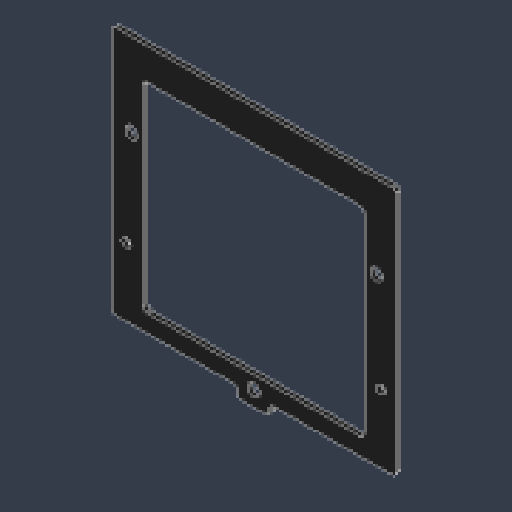
# Autodesk Inventor part: PlacementTest
Saved by Autodesk Inventor 2023.4 (Build 274418000, 418)
## iProperties
Created: 2024-02-22
Part Number: PlacementTest
Material: Generic
Document SubType Name: Modeling
Designer: JoaoSilva
Density: 1 g/cm^3
Appearance: Smooth - Black
Author: JoaoSilva
Autodesk Inventor part; units mm, degrees
ref_plane "YZ Plane" through (0, 0, 0) normal (1, 0, 0) x (0, 1, 0)
ref_plane "XZ Plane" through (0, 0, 0) normal (0, 1, 0) x (-1, 0, 0)
ref_plane "XY Plane" through (0, 0, 0) normal (0, 0, 1) x (1, 0, 0)
sketch "Sketch1" plane through (0, 0, 0) normal (0, 0, 1) x (1, 0, 0)
  line L0 (-40, 32.5) -> (40, 32.5)
  line L1 (40, 32.5) -> (40, -32.5)
  line L2 (40, -32.5) -> (-40, -32.5)
  line L3 (-40, -32.5) -> (-40, 32.5)
  line L4 (-40, 32.5) -> (40, -32.5) construction
  line L5 (40, 32.5) -> (-40, -32.5) construction
  line L6 (-8, 32.5) -> (-8, 24.5)
  line L7 (-8, 24.5) -> (-20, 24.5)
  line L8 (-20, 24.5) -> (-20, 28.5)
  line L9 (-20, 28.5) -> (-40, 28.5)
  line L10 (-40, -27) -> (-19, -27)
  line L11 (-19, -27) -> (-15.5, -23.5)
  line L12 (-15.5, -23.5) -> (-9.5, -23.5)
  line L13 (-9.5, -23.5) -> (-9.5, -32.5)
  line L14 (9.5, -32.5) -> (9.5, -23.5)
  line L15 (9.5, -23.5) -> (15.5, -23.5)
  line L16 (15.5, -23.5) -> (19, -27)
  line L17 (19, -27) -> (40, -27)
  point P0 (0, 0)
  dimension "d0" = 80
  dimension "d1" = 65
  dimension "d2" = 19
  dimension "d3" = 45
  dimension "d4" = 9
  dimension "d5" = 3.5
  dimension "d6" = 6
  dimension "d7" = 45
  dimension "d8" = 8
  dimension "d9" = 8
  dimension "d10" = 12
  dimension "d11" = 4
  constraints: 36 end point, 9 perpendicular, 6 point on line, 4 equal length, 3 parallel, 2 midpoint, 1 horizontal, 1 vertical
  measures "d0" distance of L1.end L2.end
  measures "d1" distance of L0.end L1.end
  measures "d2" distance between parallel lines of L14 L13
  measures "d3" angle of L10 L11
  measures "d4" distance of L12.end L13.end
  measures "d5" distance between parallel lines of L12 L10
  measures "d6" distance of L11.end L12.end
  measures "d7" angle of L17 L16
  measures "d8" distance from line of point (0, 0) L6
  measures "d9" distance of L6.start L6.end
  measures "d10" distance of L6.end L7.end
  measures "d11" distance between parallel lines of L7 L9
extrude "Extrusion1" add sketch "Sketch1" along normal blind 1.3 contours L0 L1 L17 L16 L15 L14 L2 L13 L12 L11 L10 L3 L9 L8 L7 L6
sketch "Sketch2" plane through (0, 0, 1.3) normal (0, 0, 1) x (1, 0, 0)
  line L0 (-35.7, -4.3) -> (35.7, -4.3) construction
  line L1 (-40, -27) -> (-19, -27) projected
  point P0 (0, 0)
  point P1 (0, -4.3)
  dimension "d14" = 71.4
  dimension "d15" = 22.7
  constraints: 2 end point, 1 horizontal, 1 midpoint, 1 vertical alignment
  measures "d14" distance of L0.start L0.end
  measures "d15" distance between parallel lines of L1 L0
hole "Hole1" at (-35.7, -4.3, 1.3) at (35.7, -4.3, 1.3) direction (0, 0, -1) diameter 2.5 end through all
sketch "Sketch4" plane through (-8, 32.5, 0) normal (0, 1, 0) x (1, 0, 0)
  line L0 (10.9, -2.9) -> (5.1, -2.9) construction
  line L1 (10.9, -1.3) -> (5.1, -1.3)
  line L2 (5.1, -4.5) -> (10.9, -4.5)
  arc A0 (10.9, -4.5) -> (10.9, -1.3) centre (10.9, -2.9) ccw
  arc A1 (5.1, -1.3) -> (5.1, -4.5) centre (5.1, -2.9) ccw
  line L3 (48, -1.3) -> (0, -1.3) projected
  line L4 (10.9, -2.9) -> (5.1, -2.9) construction
  line L5 (10.9, -1.7) -> (5.1, -1.7)
  line L6 (5.1, -4.1) -> (10.9, -4.1)
  arc A2 (10.9, -4.1) -> (10.9, -1.7) centre (10.9, -2.9) ccw
  arc A3 (5.1, -1.7) -> (5.1, -4.1) centre (5.1, -2.9) ccw
  point P0 (8, 0)
  point P1 (8, -2.9)
  point P2 (3.5, -2.9)
  point P3 (12.5, -2.9)
  point P4 (8, -2.9)
  dimension "d23" = 3.2
  dimension "d24" = 9
  dimension "d25" = 0.4
  constraints: 16 end point, 10 point on circle, 8 tangent, 4 centre point, 3 equal length, 2 midpoint, 1 collinear, 1 horizontal, 1 vertical alignment
  measures "d23" distance between parallel lines of L2 L1
  measures "d24" distance of point (3.5, -2.9) point (12.5, -2.9)
  measures "d25" distance between parallel lines of L2 L6
extrude "Extrusion2" add sketch "Sketch4" against normal blind 6.8
sketch "Sketch5" plane through (0, 0, 1.3) normal (0, 0, 1) x (1, 0, 0)
  circle A0 centre (-34.4, 23.1) radius 1.7
  circle A1 centre (34.4, 23.1) radius 1.7
  circle A2 centre (0, -22.3) radius 1.7
  line L0 (-34.4, 23.1) -> (34.4, 23.1) construction
  circle A3 centre (35.7, -4.3) radius 1.25 projected
  point P0 (0, 0)
  point P1 (0, 23.1)
  dimension "d28" = 3.4
  dimension "d29" = 68.8
  dimension "d30" = 27.4
  dimension "d31" = 18
  constraints: 3 centre point, 2 end point, 2 equal radius, 2 vertical alignment, 1 horizontal, 1 horizontal alignment, 1 midpoint
  measures "d28" diameter of A2
  measures "d29" distance of L0.start L0.end
  measures "d30" distance from line of A3.centre L0
  measures "d31" vertical distance of A3.centre A2.centre
extrude "Extrusion3" add sketch "Sketch5" along normal blind 0.4 contours A0 | A1 | A2
sketch "Sketch6" plane through (0, -22.3, 1.7) normal (0, 0, 1) x (1, 0, 0)
  circle A0 centre (0, 0) radius 1.7 projected
  circle A1 centre (-34.4, 45.4) radius 1.7 projected
  circle A2 centre (34.4, 45.4) radius 1.7 projected
  point P0 (0, 22.3)
extrude "Extrusion4" cut sketch "Sketch6" against normal through all
sketch "Sketch7" plane through (0, 0, 1.3) normal (0, 0, 1) x (1, 0, 0)
  line L0 (40, 32.5) -> (-8, 32.5) projected
  line L1 (40, 32.5) -> (40, 46.5)
  line L2 (40, 46.5) -> (-40, 46.5)
  line L3 (-40, 28.5) -> (-40, -27) projected
  line L4 (-40, 46.5) -> (-40, 28.5)
  line L5 (-40, 28.5) -> (-31, 28.5)
  line L6 (-20, 28.5) -> (-40, 28.5) projected
  line L7 (-31, 28.5) -> (-31, 37.5)
  line L8 (-31, 37.5) -> (31, 37.5)
  line L9 (31, 37.5) -> (31, 32.5)
  point P0 (0, 0)
  dimension "d36" = 9
  dimension "d37" = 9
  dimension "d38" = 9
  dimension "d39" = 5
  constraints: 14 end point, 4 perpendicular, 2 point on line, 2 vertical
  measures "d36" distance between parallel lines of L7 L4
  measures "d37" distance between parallel lines of L2 L8
  measures "d38" distance between parallel lines of L1 L9
  measures "d39" distance between parallel lines of L0 L8
extrude "Extrusion5" add sketch "Sketch7" against normal up to surface (1.3 mm away)
sketch "Sketch8" plane through (0, 0, 1.3) normal (0, 0, 1) x (1, 0, 0)
  line L0 (31, 32.5) -> (2.9, 32.5) projected
  line L1 (31, 32.5) -> (-31, 32.5)
  line L2 (-31, 32.5) -> (-31, -18.5)
  line L3 (-31, -18.5) -> (31, -18.5)
  line L4 (31, -18.5) -> (31, 32.5)
  line L5 (-31, 28.5) -> (-31, 37.5) projected
  line L6 (-15.5, -23.5) -> (-9.5, -23.5) projected
  line L7 (-40, -27) -> (-19, -27) projected
  line L8 (-15.5, -23.5) -> (-40, -23.5)
  line L9 (-40, -23.5) -> (-40, -27)
  line L10 (-40, -27) -> (-15.5, -27)
  line L11 (-15.5, -27) -> (-15.5, -23.5)
  line L12 (15.5, -23.5) -> (19, -27) projected
  line L13 (19, -27) -> (40, -27) projected
  line L14 (15.5, -23.5) -> (40, -23.5)
  line L15 (40, -23.5) -> (40, -27)
  line L16 (40, -27) -> (15.5, -27)
  line L17 (15.5, -27) -> (15.5, -23.5)
  line L18 (9.5, -32.5) -> (9.5, -23.5) projected
  line L19 (-9.5, -32.5) -> (9.5, -32.5) projected
  line L20 (9.5, -26.5) -> (-9.5, -26.5)
  line L21 (-9.5, -26.5) -> (-9.5, -32.5)
  line L22 (-9.5, -32.5) -> (9.5, -32.5)
  line L23 (9.5, -32.5) -> (9.5, -26.5)
  line L24 (-9.5, -23.5) -> (-9.5, -32.5) projected
  line L25 (-9.5, -23.5) -> (-4.5, -23.5)
  line L26 (-4.5, -23.5) -> (-4.5, -26.5)
  line L27 (-4.5, -26.5) -> (-9.5, -26.5)
  line L28 (-9.5, -26.5) -> (-9.5, -23.5)
  line L29 (9.5, -23.5) -> (15.5, -23.5) projected
  line L30 (9.5, -23.5) -> (4.5, -23.5)
  line L31 (4.5, -23.5) -> (4.5, -26.5)
  line L32 (4.5, -26.5) -> (9.5, -26.5)
  line L33 (9.5, -26.5) -> (9.5, -23.5)
  point P0 (0, 0)
  point P1 (-19, -27)
  point P2 (2.9, 32.5)
  dimension "d42" = 51
  dimension "d43" = 8
  dimension "d44" = 5
  dimension "d45" = 5
  constraints: 48 end point, 12 parallel, 6 horizontal, 6 perpendicular, 3 point on line, 1 collinear
  measures "d42" distance of L1.end L2.end
  measures "d43" distance between parallel lines of L3 L20
  measures "d44" distance of L18.end L30.end
  measures "d45" distance of L6.end L25.end
extrude "Extrusion6" cut sketch "Sketch8" against normal through all
sketch "Sketch9" plane through (-2.9, 32.5, 4.5) normal (0, 0, 1) x (1, 0, 0)
  line L0 (-5.3856, 3.3152) -> (10.2234, 3.3152)
  line L1 (10.2234, 3.3152) -> (10.2234, -11.8662)
  line L2 (10.2234, -11.8662) -> (-5.3856, -11.8662)
  line L3 (-5.3856, -11.8662) -> (-5.3856, 3.3152)
  point P0 (2.9, -32.5)
  constraints: 8 end point, 2 parallel, 1 horizontal, 1 perpendicular
extrude "Extrusion7" cut sketch "Sketch9" against normal through all
fillet "Fillet1" radius 1 12 edges at (-31, 37.5, 0.65) (-40, 46.5, 0.65) (31, 37.5, 0.65) (40, 46.5, 0.65) (40, -23.5, 0.65) (31, -18.5, 0.65) (4.5, -23.5, 0.65) (4.5, -26.5, 0.65) (-4.5, -26.5, 0.65) (-4.5, -23.5, 0.65) (-31, -18.5, 0.65) (-40, -23.5, 0.65)
equation "\"d7\" = d3"
equation "\"d37\" = d36"
equation "\"d38\" = d36"
equation "\"d45\" = d44"
body "Solid1"
